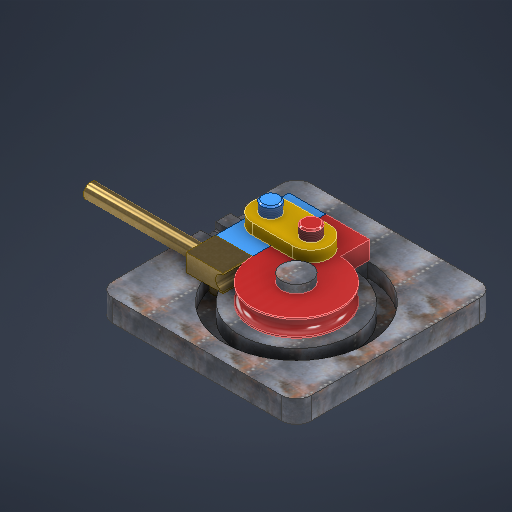
# Autodesk Inventor part: Part1
Saved by Autodesk Inventor 2026.1 (Build 301233020, 233B)
## iProperties
Created: 2025-12-25
Part Number: Part1
Material: Generic
Document SubType Name: Modeling
Designer: kngob
Density: 1 g/cm^3
Appearance: Default
Author: kngob
Autodesk Inventor part; units mm, degrees
ref_plane "YZ Plane" through (0, 0, 0) normal (1, 0, 0) x (0, 1, 0)
ref_plane "XZ Plane" through (0, 0, 0) normal (0, 1, 0) x (-1, 0, 0)
ref_plane "XY Plane" through (0, 0, 0) normal (0, 0, 1) x (1, 0, 0)
sketch "Sketch1" plane through (0, 0, 0) normal (0, 0, 1) x (1, 0, 0)
  line L0 (-110, 12) -> (0, 12)
  line L1 (0, 12) -> (0, -12)
  line L2 (0, -12) -> (-110, -12)
  line L3 (-110, -12) -> (-110, 12)
  circle A0 centre (-60, 0) radius 10
  line L4 (-60, 12) -> (-60, 10)
  line L5 (-60, -10) -> (-60, -12)
  point P0 (0, 0)
  point P1 (0, 0)
  dimension "d0" = 110
  dimension "d1" = 24
  dimension "d3" = 20
  dimension "d4" = 2
  dimension "d5" = 2
  dimension "d6" = 60
  constraints: 12 end point, 3 perpendicular, 2 point on circle, 2 point on line, 1 centre point, 1 coincident, 1 collinear, 1 horizontal, 1 midpoint, 1 parallel
  measures "d0" distance of L0.start L0.end
  measures "d1" distance of L0.end L1.end
  measures "d3" diameter of A0
  measures "d4" distance of L4.start L4.end
  measures "d5" distance of L5.start L5.end
  measures "d6" distance between parallel lines of L1 L4
revolve "Revolution1" add sketch "Sketch1" angle 360 about axis through (0, 12, 0) along (0, -1, 0) contours L0 L1 L2 L5 A0 L4
extrude "Extrusion1" add sketch "Sketch1" against normal blind 100 contours L0 L1 L2 L5 A0 L4
extrude "Extrusion2" add sketch "Sketch1" against normal blind 100 separate body contours L0 L4 A0 L5 L2 L3
extrude "Extrusion3" add sketch "Sketch1" along normal blind 40 separate body contours L0 L4 A0 L5 L2 L3
sketch "Sketch2" plane through (-60, 12, -100) normal (0, 1, 0) x (1, 0, 0)
  circle A0 centre (60, -100) radius 20
  dimension "d14" = 40
  constraints: 1 centre point, 1 coincident
  measures "d14" diameter of A0
extrude "Extrusion4" cut sketch "Sketch2" against normal blind 40 bodies 1
sketch "Sketch3" plane through (-110, -12, 0) normal (-1, 0, 0) x (0, 0, 1)
  line L0 (0, 0) -> (-100, 0) projected
  line L1 (-80, 0) -> (-60, 0)
  line L2 (-60, 0) -> (-60, -10)
  line L3 (-60, -10) -> (-80, -10)
  line L4 (-80, -10) -> (-80, 0)
  line L5 (-40, 0) -> (-20, 0)
  line L6 (-20, 0) -> (-20, -10)
  line L7 (-20, -10) -> (-40, -10)
  line L8 (-40, -10) -> (-40, 0)
  line L9 (-60, -10) -> (-40, -10) construction
  line L10 (0, 24) -> (-100, 24) projected
  point P0 (0, 12)
  point P1 (-50, -10)
  point P2 (-50, 24)
  dimension "d17" = 20
  dimension "d18" = 10
  dimension "d19" = 20
  constraints: 18 end point, 4 parallel, 3 horizontal, 3 point on line, 2 midpoint, 2 perpendicular, 1 collinear, 1 vertical alignment
  measures "d17" distance of L2.end L3.end
  measures "d18" distance of L1.end L2.end
  measures "d19" distance of L2.end L7.end
extrude "Extrusion5" add sketch "Sketch3" against normal up to surface (50 mm away) bodies 2
fillet "Fillet1" radius 2 4 edges at (-85, -22, -80) (-85, -22, -60) (-85, -22, -40) (-85, -22, -20)
sketch "Sketch4" plane through (-110, -12, 0) normal (-1, 0, 0) x (0, 0, 1)
  line L0 (20, 24) -> (20, 0) projected
  circle A0 centre (20, 12) radius 10
  line L1 (40, 24) -> (40, 0) projected
  line L2 (0, 24) -> (40, 24) projected
  point P0 (0, 12)
  point P1 (40, 12)
  point P2 (20, 24)
  dimension "d23" = 20
  constraints: 3 midpoint, 1 centre point, 1 horizontal alignment, 1 vertical alignment
  measures "d23" diameter of A0
extrude "Extrusion6" add sketch "Sketch4" along normal blind 150 bodies 3
sketch "Sketch5" plane through (-110, -12, 0) normal (0, -1, 0) x (1, 0, 0)
  circle A0 centre (25, 20) radius 10
  line L0 (0, 40) -> (50, 40) projected
  line L1 (0, 0) -> (0, 40) projected
  point P0 (110, 0)
  point P1 (25, 40)
  point P2 (0, 20)
  dimension "d26" = 20
  constraints: 2 midpoint, 1 centre point, 1 horizontal alignment, 1 vertical alignment
  measures "d26" diameter of A0
extrude "Extrusion7" add sketch "Sketch5" along normal blind 20 bodies 3
fillet "Fillet2" radius 2 1 edges at (-95, -32, 20)
sketch "Sketch6" plane through (-60, 12, -100) normal (0, 1, 0) x (1, 0, 0)
  circle A0 centre (30, -50) radius 12.5
  line L0 (-50, -100) -> (-50, 0) projected
  line L1 (0, 0) -> (60, 0) projected
  point P0 (60, -100)
  point P1 (-50, -50)
  point P2 (30, 0)
  dimension "d30" = 25
  constraints: 2 midpoint, 1 centre point, 1 horizontal alignment, 1 vertical alignment
  measures "d30" diameter of A0
extrude "Extrusion8" add sketch "Sketch6" along normal blind 30 bodies 1
sketch "Sketch7" plane through (-110, 12, 0) normal (0, 1, 0) x (1, 0, 0)
  circle A0 centre (25, 50) radius 12.5
  line L0 (0, 0) -> (0, 100) projected
  line L1 (0, 100) -> (50, 100) projected
  point P0 (110, 0)
  point P1 (0, 50)
  point P2 (25, 100)
  dimension "d33" = 25
  constraints: 2 midpoint, 1 centre point, 1 horizontal alignment, 1 vertical alignment
  measures "d33" diameter of A0
extrude "Extrusion9" add sketch "Sketch7" along normal blind 30 bodies 2
thread "Thread3" size "M25x2" class "6g" standard "ANSI Metric M Profile" length 20 offset 10
thread "Thread4" size "M25x2" class "6g" standard "ANSI Metric M Profile" length 20
sketch "Sketch8" plane through (-60, 12, -100) normal (0, 1, 0) x (1, 0, 0)
  circle A0 centre (-25, -50) radius 12.5 projected
  circle A1 centre (30, -50) radius 12.5 projected
  line L0 (-25, -50) -> (30, -50) construction
  line L1 (-25, -75) -> (30, -75)
  line L2 (30, -25) -> (-25, -25)
  arc A2 (-25, -25) -> (-25, -75) centre (-25, -50) ccw
  arc A3 (30, -75) -> (30, -25) centre (30, -50) ccw
  point P0 (60, -100)
  point P1 (2.5, -50)
  dimension "d44" = 25
  constraints: 8 end point, 4 point on circle, 4 tangent, 2 centre point, 1 horizontal, 1 midpoint, 1 parallel
  measures "d44" radius of A3
extrude "Extrusion10" add sketch "Sketch8" along normal blind 15 separate body
chamfer "Chamfer1" distance 2 angle 45 2 edges at (-42.5, 42, -50) (-97.5, 42, -50)
sketch "Sketch9" plane through (-60, -12, -100) normal (0, -1, 0) x (1, 0, 0)
  line L0 (160, 220) -> (-70, 220)
  line L1 (-90, 200) -> (-90, -30)
  line L2 (-70, -50) -> (160, -50)
  line L3 (180, -30) -> (180, 200)
  arc A0 (-70, 220) -> (-90, 200) centre (-70, 200) ccw
  arc A1 (180, 200) -> (160, 220) centre (160, 200) ccw
  arc A2 (160, -50) -> (180, -30) centre (160, -30) ccw
  arc A3 (-90, -30) -> (-70, -50) centre (-70, -30) ccw
  point P0 (60, 100)
  dimension "d50" = 120
  dimension "d51" = 150
  dimension "d52" = 120
  dimension "d53" = 150
  dimension "d54" = 20
  constraints: 8 end point, 8 point on circle, 8 tangent, 4 centre point, 3 equal radius, 2 parallel, 1 horizontal, 1 perpendicular
  measures "d50" distance from line of L3 point (60, 100)
  measures "d51" distance from line of L1 point (60, 100)
  measures "d52" distance from line of point (60, 100) L0
  measures "d53" distance from line of L2 point (60, 100)
  measures "d54" radius of A0
extrude "Extrusion11" add sketch "Sketch9" along normal blind 30 separate body
sketch "Sketch10" plane through (-150, -12, -130) normal (-1, 0, 0) x (0, 0, 1)
  arc A0 (108, -10) -> (110, -8) centre (108, -8) ccw projected
  line L0 (110, -8) -> (110, 0) projected
  line L1 (130, 0) -> (110, 0) projected
  line L2 (130, 24) -> (130, 0) projected
  line L3 (130, 24) -> (30, 24) projected
  line L4 (30, 0) -> (30, 24) projected
  line L5 (50, 0) -> (30, 0) projected
  line L6 (50, 0) -> (50, -8) projected
  arc A1 (50, -8) -> (52, -10) centre (52, -8) ccw projected
  line L7 (52, -10) -> (68, -10) projected
  arc A2 (68, -10) -> (70, -8) centre (68, -8) ccw projected
  line L8 (70, -8) -> (70, 0) projected
  line L9 (90, 0) -> (70, 0) projected
  line L10 (90, 0) -> (90, -8) projected
  arc A3 (90, -8) -> (92, -10) centre (92, -8) ccw projected
  line L11 (92, -10) -> (108, -10) projected
  line L12 (230, 0) -> (0, 0) projected
  point P0 (130, 12)
extrude "Extrusion12" cut sketch "Sketch10" against normal up to surface (90 mm away) contours L11 A3 L10 L12 L0 A0 | L8 A2 L7 A1 L6 L12 bodies 5
sketch "Sketch11" plane through (-60, -12, -100) normal (0, 1, 0) x (1, 0, 0)
  circle A0 centre (60, -100) radius 20 projected
extrude "Extrusion13" add sketch "Sketch11" along normal blind 35 bodies 5
sketch "Sketch12" plane through (-60, -12, -100) normal (0, 1, 0) x (1, 0, 0)
  circle A0 centre (-25, -120) radius 10 construction
  arc A1 (-37.3212, -100) -> (60, -2.6788) centre (60, -100) ccw
  arc A2 (-17.3212, -100) -> (60, -22.6788) centre (60, -100) ccw
  line L0 (60, -100) -> (-37.3212, -100)
  line L1 (60, -100) -> (60, -2.6788)
  constraints: 4 end point, 4 point on circle, 2 centre point, 2 coincident, 2 point on line, 2 tangent, 1 horizontal, 1 perpendicular
extrude "Extrusion14" cut sketch "Sketch12" against normal blind 20 contours L0 A2 L1 A1 bodies 5
